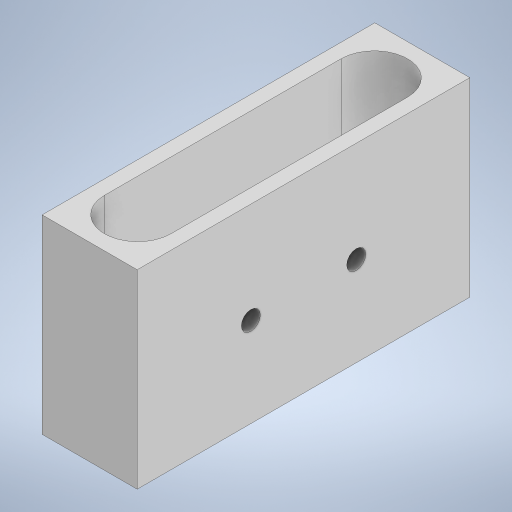
# Autodesk Inventor part: ResonantSlider
Saved by Autodesk Inventor 2023 (Build 270158000, 158)
## iProperties
Created: 2024-01-12
Part Number: ResonantSlider
Material: Generic
Document SubType Name: Modeling
Designer: kerlin
Density: 1 g/cm^3
Appearance: Default
Author: kerlin
Autodesk Inventor part; units mm, degrees
ref_plane "YZ Plane" through (0, 0, 0) normal (1, 0, 0) x (0, 1, 0)
ref_plane "XZ Plane" through (0, 0, 0) normal (0, 1, 0) x (-1, 0, 0)
ref_plane "XY Plane" through (0, 0, 0) normal (0, 0, 1) x (1, 0, 0)
sketch "Sketch1" plane through (0, 0, 0) normal (0, 1, 0) x (-1, 0, 0)
  line L0 (5, -12.5) -> (-5, -12.5)
  line L1 (-5, -12.5) -> (-5, 12.5)
  line L2 (-5, 12.5) -> (5, 12.5)
  line L3 (5, 12.5) -> (5, -12.5)
  line L4 (5, -12.5) -> (-5, 12.5) construction
  line L5 (-5, -12.5) -> (5, 12.5) construction
  point P0 (0, 0)
  dimension "d0" = 10
  dimension "d1" = 25
  constraints: 12 end point, 2 midpoint, 2 parallel, 1 horizontal, 1 perpendicular
  measures "d0" distance of L1.end L2.end
  measures "d1" distance of L0.end L1.end
extrude "Extrusion1" add sketch "Sketch1" along normal blind 20
sketch "Sketch2" plane through (5, 0, 12.5) normal (1, 0, 0) x (0, 0, -1)
  line L0 (0, 0) -> (25, 0) projected
  line L1 (0, 0) -> (0, 20) projected
  point P0 (12.5, 0)
  point P1 (6.9565, 9.4)
  point P2 (18.0435, 9.4)
  dimension "d11" = 9.4
  dimension "d12" = 9.4
  dimension "d13" = 11.087
  dimension "d14" = 6.9565
  measures "d11" distance from line of L0 point (6.957, 9.4)
  measures "d12" distance from line of L0 point (18.044, 9.4)
  measures "d13" distance of point (18.044, 9.4) point (6.957, 9.4)
  measures "d14" distance from line of L1 point (6.957, 9.4)
hole "Hole1" at (5, 9.4, 5.5435) at (5, 9.4, -5.5435) direction (-1, 0, 0) diameter 2 depth 25
sketch "Sketch3" plane through (5, 0, -12.5) normal (0, 0, -1) x (-1, 0, 0)
  line L0 (0, 0) -> (0, 20) projected
  line L1 (10, 0) -> (10, 20) projected
  line L2 (0, 20) -> (10, 20)
  line L3 (10, 20) -> (10, 0)
  line L4 (10, 0) -> (0, 0)
  line L5 (0, 0) -> (0, 20)
  point P0 (5, 0)
  constraints: 8 end point, 2 parallel, 1 horizontal, 1 perpendicular
extrude "Extrusion2" add sketch "Sketch3" along normal blind 5
sketch "Sketch4" plane through (-5, 0, 12.5) normal (0, 0, 1) x (1, 0, 0)
  line L0 (0, 0) -> (0, 20) projected
  line L1 (10, 0) -> (0, 0)
  line L2 (0, 0) -> (0, 20)
  line L3 (0, 20) -> (10, 20)
  line L4 (10, 20) -> (10, 0)
  point P0 (5, 0)
  constraints: 8 end point, 2 parallel, 1 horizontal, 1 perpendicular
extrude "Extrusion3" add sketch "Sketch4" along normal blind 5
sketch "Sketch5" plane through (0, 20, 0) normal (0, 1, 0) x (1, 0, 0)
  line L0 (0, -15.9498) -> (0, 15.9498) construction
  line L1 (3.5, -12.4498) -> (3.5, 12.4498)
  line L2 (-3.5, 12.4498) -> (-3.5, -12.4498)
  arc A0 (-3.5, -12.4498) -> (3.5, -12.4498) centre (0, -12.4498) ccw
  arc A1 (3.5, 12.4498) -> (-3.5, 12.4498) centre (0, 12.4498) ccw
  point P0 (0, 0)
  point P1 (0, 0)
  dimension "d19" = 7
  constraints: 8 end point, 6 point on circle, 4 tangent, 2 centre point, 2 point on line, 1 midpoint, 1 parallel, 1 vertical
  measures "d19" diameter of A1
extrude "Extrusion4" cut sketch "Sketch5" against normal blind 17
sketch "Sketch6" plane through (0, 3, 0) normal (0, 1, 0) x (1, 0, 0)
  line L0 (0, -13.8879) -> (0, 14.164) construction
  line L1 (2, -11.8879) -> (2, 12.164)
  line L2 (-2, 12.164) -> (-2, -11.8879)
  arc A0 (-2, -11.8879) -> (2, -11.8879) centre (0, -11.8879) ccw
  arc A1 (2, 12.164) -> (-2, 12.164) centre (0, 12.164) ccw
  point P0 (0, 0)
  point P1 (0, 0.1381)
  dimension "d22" = 4
  constraints: 8 end point, 6 point on circle, 4 tangent, 2 centre point, 2 point on line, 1 midpoint, 1 parallel, 1 vertical
  measures "d22" diameter of A1
extrude "Extrusion5" cut sketch "Sketch6" against normal blind 15
body "Solid1"
